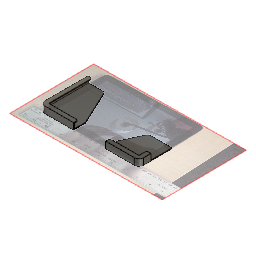
Fire_Tablet_HD_8_2024_Release_Wall_Bracket (Autodesk Fusion 360 design; units mm, degrees)
Autodesk Fusion 360 part; units mm, degrees
note: some values were not read from the file. Set by a fixed rule: which sketch regions a step uses.
sketch "Sketch3" plane through (0, 0, 0) normal (0, 0, 1) x (1, 0, 0)
  line L0 (-119.6649, -54.162) -> (-59.7, -54.162)
  line L1 (-59.7, -54.162) -> (-59.7, -29.162)
  line L2 (-94.7, 45.838) -> (-129.7, 45.838)
  line L3 (-129.7, 45.838) -> (-129.7, -44.4306)
  arc A0 (-129.7, -44.4306) -> (-119.6649, -54.162) centre (-119.6649, -44.1221) ccw
  line L4 (-127.7, 45.838) -> (-127.7, -44.3981)
  arc A1 (-127.7, -44.3981) -> (-119.6649, -52.162) centre (-119.6649, -44.1221) ccw
  line L5 (-119.6649, -52.162) -> (-59.7, -52.162)
  line L6 (-94.7, 45.838) -> (-59.7, -29.162)
  dimension "d5" = -2
  constraint horizontal L0
  constraint vertical L1
  constraint horizontal L2
  constraint vertical L3
  constraint tangent L0 A0
extrude "Extrude1" add sketch "Sketch3" along normal blind 2 contours L1 L2 L4 A1 L5 L6 makes body 1
extrude "Extrude2" add sketch "Sketch3" along normal blind 12 contours L0 L1 L2 L3 A0 L4 A1 L5 bodies 1
ref_plane "WorkPlane1" through (-94.7, -4.162, 12) normal (0, 0, 1) x (1, 0, 0)
sketch "Sketch5" plane through (0, 0, 12) normal (0, 0, 1) x (1, 0, 0)
  arc A0 (-127.7, -44.3981) -> (-119.6649, -52.162) centre (-119.6649, -44.1221) ccw
  line L0 (-127.7, -44.3981) -> (-127.7, 45.838)
  line L1 (-59.7, -52.162) -> (-119.6649, -52.162)
  line L2 (-129.7, 45.838) -> (-129.7, -44.4306)
  arc A1 (-129.7, -44.4306) -> (-119.6649, -54.162) centre (-119.6649, -44.1221) ccw
  line L3 (-119.6649, -54.162) -> (-59.7, -54.162)
  line L4 (-59.7, -54.162) -> (-59.7, -52.162)
  line L5 (-127.7, 45.838) -> (-129.7, 45.838)
  line L6 (-129.7, 45.838) -> (-129.7, -44.4306)
  line L7 (-59.7, -54.162) -> (-119.6649, -54.162)
  arc A2 (-129.7, -44.4306) -> (-119.6649, -54.162) centre (-119.6649, -44.1221) ccw
  line L8 (-59.7, -45.162) -> (-119.6649, -45.162)
  line L9 (-120.7, 45.838) -> (-120.7, -44.4306)
  line L10 (-59.7, -45.162) -> (-59.7, -54.162)
  line L11 (-120.7, 45.838) -> (-129.7, 45.838)
  arc A3 (-120.7, -44.4306) -> (-119.6649, -45.162) centre (-119.6649, -44.0638) ccw
  line L12 (-120.7, 45.838) -> (-120.7, 42.3306)
  dimension "d11" = 9
  dimension "d12" = -9
  constraint coincident L2.start L5.end
  constraint coincident L2.end A1.start
  constraint coincident L3.end L4.start
  constraint coincident A1.end L3.start
  constraint tangent L3 A2
  constraint perpendicular L3 L10
  constraint perpendicular L2 L11
  constraint tangent L8 A3
  constraint coincident L9 L12.end
extrude "Extrude3" add sketch "Sketch5" along normal blind 2 bodies 1
fillet "Fillet1" radius 3 1 edges at (-120.7, 45.838, 13) on bodies 1
fillet "Fillet2" radius 3 1 edges at (-59.7, -45.162, 13) on bodies 1
fillet "Fillet3" radius 7 1 edges at (-94.7, 45.838, 1) on bodies 1
fillet "Fillet4" radius 3 1 edges at (-59.7, -29.162, 1) on bodies 1
mirror "Mirror1" about plane through (0, 0, 0) normal (1, 0, 0) of bodies 1 makes body 2
move_body "Move2" bodies 2 to x (1, 0, 0) y (0, 1, 0) z (0, 0, 1) at (-52.6012, 0, 0)
sketch "Sketch6" plane through (0, 0, 12) normal (0, 0, 1) x (1, 0, 0)
  line L0 (23.1586, 15.3095) -> (88.2823, 15.3095)
  line L1 (88.2823, 15.3095) -> (88.2823, 53.2336)
  line L2 (88.2823, 53.2336) -> (23.1586, 53.2336)
  line L3 (23.1586, 53.2336) -> (23.1586, 15.3095)
  constraint horizontal L0
  constraint vertical L1
  constraint horizontal L2
  constraint vertical L3
extrude "Extrude4" cut sketch "Sketch6" along normal mid plane 63.968 bodies 2
ref_plane "WorkPlane2" through (77.0988, -14.5605, 7) normal (1, 0, 0) x (0, -1, 0)
sketch "Sketch7" plane through (77.0988, 0, 0) normal (1, 0, 0) x (0, 1, 0)
  line L0 (15.3095, 14) -> (15.3095, 12)
  line L1 (15.3095, 2) -> (15.3095, 0)
  line L2 (15.3095, 12) -> (15.3095, 2)
  line L3 (-54.162, 0) -> (-29.8276, 0)
  line L4 (-29.8276, 0) -> (-28.5589, 0)
  line L5 (15.3095, 0) -> (-28.5589, 0)
  line L6 (-44.4306, 14) -> (15.3095, 14)
  line L7 (-45.162, 14) -> (-44.4306, 14)
  line L8 (-45.162, 14) -> (-48.162, 14)
  line L9 (-54.162, 14) -> (-48.162, 14)
  line L10 (-54.162, 0) -> (-54.162, 14)
  line L11 (-54.162, 14) -> (-29.162, 14)
  line L12 (-29.162, 14) -> (-29.162, 0)
  line L13 (-29.162, 0) -> (-54.162, 0)
  line L14 (-54.162, 0) -> (-54.162, 14)
  line L15 (-29.162, 14) -> (15.3095, 14)
  line L16 (15.3095, 14) -> (15.3095, 2)
  line L17 (15.3095, 2) -> (-29.162, 2)
  line L18 (-29.162, 2) -> (-29.162, 14)
  dimension "d28" = 25
  dimension "d29" = 14
  constraint horizontal L11
  constraint vertical L12
  constraint horizontal L13
  constraint vertical L14
  constraint coincident L9.start L10.end
  constraint horizontal L15
  constraint vertical L16
  constraint horizontal L17
  constraint vertical L18
  constraint coincident L1.start L2.end
  measures "d28" distance of L9.start L11.end
  measures "d29" distance of L9.start L3.start
extrude "Extrude5" cut sketch "Sketch7" along normal mid plane 54.172 contours L0 L2 L6 L12 L15 L16 L17 L18 bodies 2
fillet "Fillet5" radius 3 1 edges at (68.0987, -29.162, 13) on bodies 2
fillet "Fillet6" radius 7 1 edges at (27.8521, 15.3095, 1) on bodies 2
named bodies: "Left", "Right"
